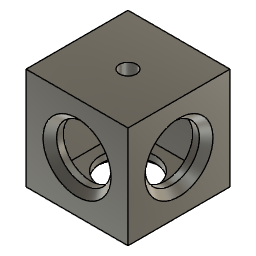
3-way cube corner connector v1 (Autodesk Fusion 360 design; units mm, degrees)
Autodesk Fusion 360 part; units mm, degrees
box "BoxPrimitive1" add length 30 width 30 height 30 placed x (0, 0, -1) y (-1, 0, 0) z (0, 1, 0) at (15, 0, 15)
shell "Shell1" thickness 4 removed faces 0 bodies 1
move_body "Move1" bodies 1 to x (1, 0, 0) y (0, 1, 0) z (0, 0, 1) at (0, -15, 0)
hole "Hole1" at (-15, 0, 0) direction (1, 0, 0) diameter 5 depth 4 tip angle 180
hole "Hole2" at (0, 0, 15) direction (0, 0, -1) diameter 5 depth 4 tip angle 180
hole "Hole3" at (0, 15, 0) direction (0, -1, 0) diameter 5 depth 4 tip angle 180
hole "Hole4" at (0, -15, 0) direction (0, 1, 0) diameter 16 depth 4 tip angle 180
hole "Hole5" at (15, 0, 0) direction (-1, 0, 0) diameter 16 depth 4 tip angle 180
hole "Hole6" at (0, 0, -15) direction (0, 0, 1) diameter 16 depth 4 tip angle 180
chamfer "Chamfer2" distance 2 angle 45 3 edges at (2.8929, -15, 7.4586) (7.4586, 2.8929, -15) (15, -7.4586, 2.8929)
